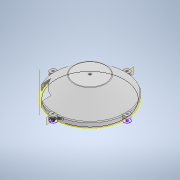
# Autodesk Inventor part: headphone_cup
Saved by Autodesk Inventor 2021 (Build 250183000, 183)
## iProperties
Created: 2021-06-10
Part Number: headphone_cup
Material: Generic
Document SubType Name: Modeling
Designer: sque793
Density: 1 g/cm^3
Appearance: Default
Author: sque793
Autodesk Inventor part; units mm, degrees
ref_plane "YZ Plane" through (0, 0, 0) normal (1, 0, 0) x (0, 1, 0)
ref_plane "XZ Plane" through (0, 0, 0) normal (0, 1, 0) x (-1, 0, 0)
ref_plane "XY Plane" through (0, 0, 0) normal (0, 0, 1) x (1, 0, 0)
sketch "Sketch1" plane through (0, 0, 0) normal (0, 1, 0) x (-1, 0, 0)
  circle A0 centre (0, 0) radius 32.2
  circle A1 centre (0, 0) radius 34.35
  circle A2 centre (0, 0) radius 33.65
  dimension "d2" = 64.4
  dimension "d3" = 68.7
  dimension "d6" = 67.3
  constraints: 3 centre point, 2 coincident
  measures "d2" diameter of A0
  measures "d3" diameter of A1
  measures "d6" diameter of A2
extrude "Extrusion2" add sketch "Sketch1" against normal blind 5.6 contours A1
sketch "Sketch2" plane through (0, 0, 0) normal (0, 1, 0) x (1, 0, 0)
  circle A0 centre (0, 0) radius 32.5
  circle A1 centre (0, 0) radius 33.65 projected
  circle A2 centre (0, 0) radius 33.65
  dimension "d9" = 65
  constraints: 2 centre point, 2 coincident, 1 concentric
  measures "d9" diameter of A0
extrude "Extrusion3" add sketch "Sketch2" against normal blind 2.6
sketch "Sketch3" plane through (0, -5.6, 0) normal (0, -1, 0) x (1, 0, 0)
  circle A0 centre (0, 0) radius 32.5 projected
  circle A1 centre (0, 0) radius 33.65 projected
  circle A2 centre (0, 0) radius 34.35 projected
  circle A3 centre (0, 0) radius 32.5 projected
  line L0 (0, 32.5) -> (0, 38.1) construction
  line L1 (0, 32.5) -> (0, 35.3) construction
  line L2 (0, 32.5) -> (0, 32.1) construction
  line L3 (0, 32.1) -> (0, 35.1) construction
  circle A4 centre (0, 35.1) radius 3
  circle A5 centre (0, 0) radius 34.35 projected
  line L4 (0, 34.35) -> (0, 35.35) construction
  circle A6 centre (0, 35.35) radius 1
  line L5 (-32.5, 0) -> (-38.1, 0) construction
  line L6 (-32.5, 0) -> (-35.3, 0) construction
  line L7 (-32.5, 0) -> (-32.1, 0) construction
  line L8 (-32.1, 0) -> (-35.1, 0) construction
  circle A7 centre (-35.1, 0) radius 3
  line L9 (-34.35, 0) -> (-35.35, 0) construction
  circle A8 centre (-35.35, 0) radius 1
  line L10 (0, -32.5) -> (0, -38.1) construction
  line L11 (0, -32.5) -> (0, -35.3) construction
  line L12 (0, -32.5) -> (0, -32.1) construction
  line L13 (0, -32.1) -> (0, -35.1) construction
  circle A9 centre (0, -35.1) radius 3
  line L14 (0, -34.35) -> (0, -35.35) construction
  circle A10 centre (0, -35.35) radius 1
  line L15 (32.5, 0) -> (38.1, 0) construction
  line L16 (32.5, 0) -> (35.3, 0) construction
  line L17 (32.5, 0) -> (32.1, 0) construction
  line L18 (32.1, 0) -> (35.1, 0) construction
  circle A11 centre (35.1, 0) radius 3
  line L19 (34.35, 0) -> (35.35, 0) construction
  circle A12 centre (35.35, 0) radius 1
  point P0 (-2.871, 34.2298)
  point P1 (-2.5696, 33.5517)
  point P2 (2.5696, 33.5517)
  point P3 (2.871, 34.2298)
  point P4 (-33.5517, 2.5696)
  point P5 (-34.2298, 2.871)
  point P6 (-34.2298, -2.871)
  point P7 (-33.5517, -2.5696)
  point P8 (-2.5696, -33.5517)
  point P9 (-2.871, -34.2298)
  point P10 (2.871, -34.2298)
  point P11 (2.5696, -33.5517)
  point P12 (33.5517, -2.5696)
  point P13 (34.2298, -2.871)
  point P14 (34.2298, 2.871)
  point P15 (33.5517, 2.5696)
  dimension "d12" = 5.6
  dimension "d14" = 0.4
  dimension "d15" = 3
  dimension "d16" = 1
  dimension "d19" = 360
  constraints: 40 end point, 12 point on line, 8 coincident, 4 midpoint, 4 vertical alignment, 2 horizontal alignment, 2 vertical, 87 other
  measures "d12" distance of L0.start L0.end
  measures "d14" distance of L0.start L2.end
  measures "d15" distance of L2.end L3.end
  measures "d16" distance of L4.start L4.end
extrude "Extrusion4" cut sketch "Sketch3" against normal up to surface (3 mm away) contours A11 A2 A1 | A1 A4 A2 | A9 A2 A1 | A1 A7 A2
sketch "Sketch4" plane through (0, -2.6, 0) normal (0, -1, 0) x (1, 0, 0)
  circle A0 centre (0, 35.1) radius 3 projected
  circle A1 centre (0, 35.35) radius 1 projected
  circle A2 centre (0, 0) radius 34.35 projected
  circle A3 centre (0, 0) radius 33.65 projected
  circle A4 centre (35.1, 0) radius 3 projected
  circle A5 centre (35.35, 0) radius 1 projected
  circle A6 centre (0, -35.1) radius 3 projected
  circle A7 centre (0, -35.35) radius 1 projected
  circle A8 centre (-35.1, 0) radius 3 projected
  circle A9 centre (-35.35, 0) radius 1 projected
  point P0 (-34.2298, 2.871)
  point P1 (-34.2298, -2.871)
  point P2 (-34.35, 0)
  point P3 (-2.871, -34.2298)
  point P4 (2.871, -34.2298)
  point P5 (0, -34.35)
  point P6 (34.2298, -2.871)
  point P7 (34.2298, 2.871)
  point P8 (34.35, 0)
  point P9 (-2.871, 34.2298)
  point P10 (0, 34.35)
  point P11 (2.871, 34.2298)
extrude "Extrusion5" add sketch "Sketch4" against normal blind 2.6 contours A0 A2 | A2 A8 | A4 A2 | A2 A6
ref_plane "Work Plane3" through (0, 0, 0) normal (1, 0, 0) x (0, 1, 0)
ref_plane "Work Plane1" through (-38.1, 0, 0) normal (-1, 0, 0) x (0, -1, 0)
ref_plane "Work Plane2" through (38.1, 0, 0) normal (1, 0, 0) x (0, 1, 0)
sketch "Sketch6" plane through (0, 0, 0) normal (1, 0, 0) x (0, 1, 0)
  line L0 (0, 32.5) -> (0, -32.5) construction
  line L1 (0, 0) -> (15, 0) construction
  line L2 (15, 0) -> (15, -15)
  line L3 (0, -32.5) -> (0, -33.75)
  line L4 (0, -33.75) -> (15, -15)
  line L5 (15, -15) -> (13.75, -15) construction
  line L6 (13.75, -15) -> (0, -32.5)
  line L7 (13.75, -15) -> (13.75, 0)
  line L8 (13.75, 0) -> (15, 0)
  dimension "d25" = 15
  dimension "d26" = 15
  dimension "d27" = 1.25
  dimension "d28" = 1.25
  constraints: 16 end point, 2 perpendicular, 1 collinear, 1 horizontal, 1 point on line, 1 vertical
  measures "d25" distance of L1.start L1.end
  measures "d26" distance of L1.end L2.end
  measures "d27" distance of L0.end L3.end
  measures "d28" distance of L2.end L5.end
revolve "Revolution1" add sketch "Sketch6" angle 360 about axis through (0, 0, 0) along (0, 1, 0)
ref_plane "Work Plane4" through (-24.2891, 0, 24.2891) normal (-0.7071068, 0, 0.7071068) x (0, -1, 0)
sketch "Sketch7" plane through (-24.2891, 0, 24.2891) normal (-0.7071068, 0, 0.7071068) x (0, -1, 0)
  line L0 (0, -32.5) -> (0, 32.5) construction
  line L1 (5.6, 21.9077) -> (5.6, -21.9077) construction
  line L2 (5.6, 0) -> (5.6, 10)
  line L3 (5.6, 10) -> (-4.4, 10)
  line L4 (-4.4, 10) -> (-4.4, -10)
  line L5 (-4.4, -10) -> (5.6, -10)
  line L6 (5.6, -10) -> (5.6, 0)
  point P0 (0, 0)
  dimension "d36" = 10
  dimension "d37" = 10
  dimension "d38" = 20
  constraints: 10 end point, 3 perpendicular, 2 point on line, 1 collinear, 1 midpoint
  measures "d36" distance of L2.start L2.end
  measures "d37" distance of L2.end L3.end
  measures "d38" distance of L3.end L4.end
extrude "Extrusion6" cut sketch "Sketch7" against normal up to next
sketch "Sketch8" plane through (0, 15, 0) normal (0, 1, 0) x (1, 0, 0)
  circle A0 centre (0, 0) radius 1.15
  point P0 (0, 0)
  dimension "d39" = 2.3
  constraints: 1 centre point, 1 coincident
  measures "d39" diameter of A0
extrude "Extrusion7" cut sketch "Sketch8" against normal through all
fillet "Fillet1" radius 1 6 edges at (0, 15, 15) (-24.2891, 0, -24.2891) (-32.9466, 0, 9.7184) (-9.7184, 0, 32.9466) (24.2891, 0, 24.2891) (24.2891, 0, -24.2891)
body "Solid2"
